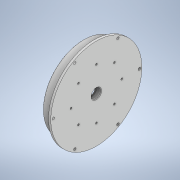
# Autodesk Inventor part: Housing_stage_output
Saved by Autodesk Inventor 2021 (Build 250183000, 183)
## iProperties
Created: 2020-05-12
Part Number: Housing_stage_output
Material: Generic
Document SubType Name: Modeling
Designer: avi41
Density: 1 g/cm^3
Appearance: Default
Author: avi41
Autodesk Inventor part; units mm, degrees
ref_plane "YZ Plane" through (0, 0, 0) normal (1, 0, 0) x (0, 1, 0)
ref_plane "XZ Plane" through (0, 0, 0) normal (0, 1, 0) x (-1, 0, 0)
ref_plane "XY Plane" through (0, 0, 0) normal (0, 0, 1) x (1, 0, 0)
sketch "Sketch1" plane through (0, 0, 0) normal (0, 1, 0) x (-1, 0, 0)
  line L0 (0, -96.425) -> (0, 8.05) construction
  line L1 (-9.27, 0) -> (22.37, 0) construction
  line L2 (-4.75, -8.5) -> (-4.75, -72.5)
  line L3 (-0.75, -72.5) -> (17.85, -72.5)
  line L4 (4.75, -58.5) -> (4.75, -8.5)
  line L5 (3.25, -8.5) -> (-4.75, -8.5)
  line L6 (4.75, -8.5) -> (4.75, -6.875)
  line L7 (4.75, -6.875) -> (3.25, -6.875)
  line L8 (3.25, -6.875) -> (3.25, -8.5)
  line L9 (17.85, -72.5) -> (17.85, -67.5777)
  line L10 (17.85, -67.5777) -> (4.5, -67.5777)
  line L11 (4.75, -58.5) -> (-1.25, -58.5)
  line L12 (-1.25, -58.5) -> (-1.25, -67.5777)
  line L13 (-1.25, -67.5777) -> (4.5, -67.5777)
  line L14 (-4.75, -72.5) -> (-4.75, -81.5)
  line L15 (-4.75, -81.5) -> (-0.75, -81.5)
  line L16 (-0.75, -81.5) -> (-0.75, -72.5)
  dimension "d7" = 8.5
  dimension "d15" = 1.5
  dimension "d18" = 1.625
  dimension "d23" = 13.1
  dimension "d25" = 64
  dimension "d26" = 6
  dimension "d27" = 50
  dimension "d28" = 4.9223
  dimension "d29" = 3.5
  dimension "d30" = 4
  dimension "d31" = 9
  constraints: 30 end point, 10 perpendicular, 4 vertical, 1 other
  measures "d7" distance between parallel lines of L1 L5
  measures "d15" distance of L6.end L7.end
  measures "d18" distance between parallel lines of L7 L5
  measures "d23" distance between parallel lines of L9 L4
  measures "d25" distance between parallel lines of L3 L5
  measures "d26" distance between parallel lines of L4 L12
  measures "d27" distance between parallel lines of L5 L11
  measures "d28" distance between parallel lines of L3 L13
  measures "d29" distance between parallel lines of L2 L12
  measures "d30" distance of L14.end L15.end
  measures "d31" distance between parallel lines of L3 L15
revolve "Revolution1" add sketch "Sketch1" angle 360 about axis through (0, 0, 0) along (-1, 0, 0)
chamfer "Chamfer1" distance 1 angle 45 1 edges at (4.75, 0, 8.5)
sketch "Sketch2" plane through (0.75, 0, 0) normal (-1, 0, 0) x (0, 0, 1)
  line L0 (0, 114.1) -> (0, -114.1) construction
  line L1 (-114.1, 0) -> (114.1, 0) construction
  circle A0 centre (0, 0) radius 72.5 projected
  circle A1 centre (0, 0) radius 81.5 projected
  circle A2 centre (0, 0) radius 77 construction
  point P0 (-77, 0)
  dimension "d33" = 4.5
  dimension "d34" = 4.5
  constraints: 1 coincident, 1 horizontal alignment, 1 point on line, 2 other
hole "Hole1" at (0.75, 0, -77) direction (1, 0, 0) diameter 4.5 end through all clearance for "Flat Head Machine Screw" size "M4" standard "Ansi Metric M Profile"
pattern_circular "Circular Pattern1" count 6 over 360 about axis through (-10, 0, 0) along (1, 0, 0) of "Hole1"
chamfer "Chamfer2" distance 0.4 angle 45 1 edges at (-17.85, 0, 72.5)
sketch "Sketch3" plane through (4.75, 0, 0) normal (1, 0, 0) x (0, 0, -1)
  line L0 (-114.1, 0) -> (114.1, 0) construction
  line L1 (0, -114.1) -> (0, 114.1) construction
  circle A0 centre (0, 0) radius 45.5 construction
  point P0 (45.5, 0)
  point P1 (32.1734, 32.1734)
  point P2 (0, 45.5)
  point P3 (-32.1734, 32.1734)
  point P4 (-45.5, 0)
  point P5 (-32.1734, -32.1734)
  point P6 (0, -45.5)
  point P7 (32.1734, -32.1734)
  dimension "d48" = 91
  dimension "d51" = 360
  constraints: 1 coincident, 1 horizontal alignment, 1 point on line, 11 other
hole "Hole2" at (4.75, 0, -45.5) at (4.75, 32.1734, -32.1734) at (4.75, 45.5, 0) at (4.75, 32.1734, 32.1734) at (4.75, 0, 45.5) at (4.75, -32.1734, 32.1734) at (4.75, -45.5, 0) at (4.75, -32.1734, -32.1734) direction (-1, 0, 0) diameter 3.242 depth 11.8 tip angle 118 thread size "M4x0.7" class "6H" standard "ANSI Metric M Profile"
equation "\"d33\" = d34"
equation "\"D_ring\" = D_ext"
equation "\"D_ext\" = 139.15534"
body "Solid1"
